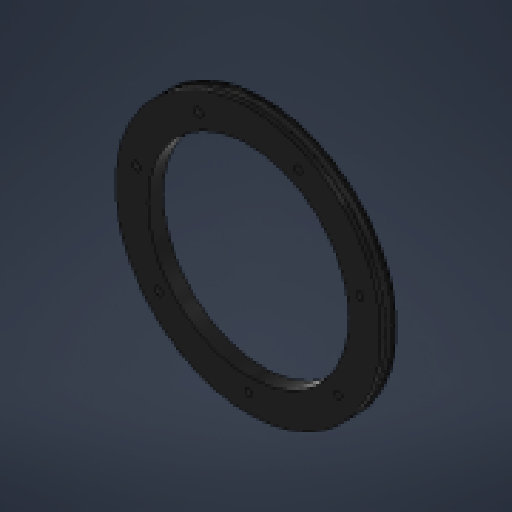
# Autodesk Inventor part: 3DPRINT,TURRET,BEARING,INNER
Saved by Autodesk Inventor 2026.1 (Build 301233020, 233B)
## iProperties
Created: 2026-02-09
Part Number: 3DPRINT,TURRET,BEARING,INNER
Material: Nylon 6/6
Document SubType Name: Modeling
Designer: littl
Density: 1.13 g/cm^3
Appearance: Smooth - Black
Mass: 187.156 g
Surface Area: 455.274 cm^2
Volume: 165.625 cm^3
Author: littl
Autodesk Inventor part; units mm, degrees
ref_plane "YZ Plane" through (0, 0, 0) normal (1, 0, 0) x (0, 1, 0)
ref_plane "XZ Plane" through (0, 0, 0) normal (0, 1, 0) x (-1, 0, 0)
ref_plane "XY Plane" through (0, 0, 0) normal (0, 0, 1) x (1, 0, 0)
sketch "Sketch1" plane through (0, 0, 0) normal (1, 0, 0) x (0, 1, 0)
  arc A0 (-107.5189, 2.6268) -> (-107.5189, -2.6268) centre (-105.3147, 0) ccw construction
  line L0 (-105.5687, 3.175) -> (-105.5687, -3.175) construction
  line L1 (-107.5189, 2.6268) -> (-107.5189, 4.635) construction
  line L2 (-106.3625, 5.1846) -> (-106.3625, 3.5971) construction
  line L3 (-107.5189, 2.6268) -> (-106.3625, 3.5971) construction
  line L4 (-107.5189, -2.6268) -> (-106.3625, -3.5971) construction
  line L5 (-131.7625, 5.1846) -> (-131.7625, -5.1846) construction
  line L6 (-131.7625, 5.1846) -> (-106.3625, 5.1846) construction
  line L7 (-131.7625, -5.1846) -> (-106.3625, -5.1846) construction
  line L8 (-106.3625, -5.1846) -> (-106.3625, -3.5971) construction
  circle A1 centre (-105.5687, 0) radius 3.175 construction
  line L9 (-35.1032, 0) -> (87.3968, 0) construction
  line L10 (-104.775, 5.1846) -> (-104.775, 3.5971)
  line L11 (-104.775, -5.1846) -> (-104.775, -3.5971)
  line L12 (-103.6186, 2.6268) -> (-104.775, 3.5971)
  line L13 (-103.6186, -2.6268) -> (-104.775, -3.5971)
  arc A2 (-103.6186, -2.6268) -> (-103.6186, 2.6268) centre (-105.8227, 0) ccw
  line L14 (-79.375, 5.1846) -> (-79.375, -5.1846)
  line L15 (0, -7.2584) -> (0, 7.2584) construction
  line L16 (-79.375, -5.1846) -> (-104.775, -5.1846)
  line L17 (-79.375, 5.1846) -> (-104.775, 5.1846) construction
  line L18 (-104.775, 5.1846) -> (-104.775, 8.5314)
  line L19 (-104.775, 8.5314) -> (-79.375, 8.5314)
  line L20 (-79.375, 8.5314) -> (-79.375, 5.1846)
  line L21 (-90.4875, 22.7342) -> (-90.4875, 8.5314) construction
  point P0 (0, 0)
  point P1 (0, 0)
  point P2 (-108.7437, 0)
  point P3 (-131.7625, 0)
  point P4 (-19.1031, 0)
  point P5 (0, 7.2584)
  point P6 (0, 0)
  point P7 (-143.7622, 15.4465)
  dimension "d0" = 6.35
  dimension "d1" = 3.429
  dimension "d2" = 50
  dimension "d3" = 1.5875
  dimension "d4" = 1.5875
  dimension "d5" = 158.75
  dimension "d7" = 25.4
  dimension "d8" = 25.4
  dimension "d9" = 180.975
  dimension "d23" = 13.716
  constraints: 42 end point, 8 point on circle, 8 symmetric about line, 5 perpendicular, 5 vertical, 4 point on line, 3 centre point, 3 midpoint, 2 collinear, 2 horizontal alignment, 2 parallel, 2 tangent, 2 vertical alignment, 1 coincident, 1 horizontal, 6 other
  measures "d0" diameter of A1
  measures "d1" radius of A0
  measures "d2" angle of L3 L1
  measures "d3" distance of L7.end L4.end
  measures "d4" distance between parallel lines of L10 L2
  measures "d7" distance of L18.end L19.end
  measures "d8" distance of L5.start L2.start
  measures "d23" distance between parallel lines of L16 L19
revolve "Revolution1" add sketch "Sketch1" angle 360 about axis through (0, 0, -7.2584) along (0, 0, 1)
sketch "Sketch2" plane through (0, 0, 8.5314) normal (0, 0, 1) x (1, 0, 0)
  point P0 (0, 0)
  point P1 (0, -90.4875)
  point P2 (70.746, -56.418)
  point P3 (88.2188, 20.1354)
  point P4 (39.2611, 81.5264)
  point P5 (-39.2611, 81.5264)
  point P6 (-88.2188, 20.1354)
  point P7 (-70.746, -56.418)
  dimension "d11" = 90.4875
  dimension "d14" = 360
  constraints: 1 vertical alignment, 8 other
  measures "d11" distance of point (0, 0) point (0, -90.487)
hole "Hole1" at (0, -90.4875, 8.5314) at (70.746, -56.418, 8.5314) at (88.2188, 20.1354, 8.5314) at (39.2611, 81.5264, 8.5314) at (-39.2611, 81.5264, 8.5314) at (-88.2188, 20.1354, 8.5314) at (-70.746, -56.418, 8.5314) direction (0, 0, -1) diameter 6.12 end through all
thicken "Thicken1" operation cut thickness 0.7937 both sides no extend neighbours no toward (0, 0, 1) faces at (-83.7461, 35.7818, -5.1846)
thicken "Thicken2" operation cut thickness 0.9656 both sides no extend neighbours no toward (0, 0, -1) faces at (-83.7461, 35.7818, 8.5314)
sketch "Sketch3" plane through (0, 0, -4.3908) normal (0, 0, -1) x (-1, 0, 0)
  line L0 (-102.1893, -8.577) -> (-91.0599, 34.4572)
  line L1 (-91.0599, 34.4572) -> (-78.7644, 31.2774)
  line L2 (-78.7644, 31.2774) -> (-89.8938, -11.7568)
  line L3 (-89.8938, -11.7568) -> (-102.1893, -8.577)
  line L4 (-102.1893, -8.577) -> (-78.7644, 31.2774) construction
  line L5 (-91.0599, 34.4572) -> (-89.8938, -11.7568) construction
  line L6 (72.9231, -53.8641) -> (84.0525, -10.83)
  line L7 (84.0525, -10.83) -> (96.3479, -14.0098)
  line L8 (96.3479, -14.0098) -> (85.2186, -57.0439)
  line L9 (85.2186, -57.0439) -> (72.9231, -53.8641)
  line L10 (72.9231, -53.8641) -> (96.3479, -14.0098) construction
  line L11 (84.0525, -10.83) -> (85.2186, -57.0439) construction
  line L12 (0, 0) -> (0, 27.097)
  point P0 (-90.4768, 11.3502)
  point P1 (84.6355, -33.9369)
  point P2 (-90.4768, 11.3502)
  point P3 (84.6355, -33.9369)
  point P4 (-90.4768, 11.3502)
  dimension "d28" = 44.45
  dimension "d29" = 12.7
  dimension "d30" = 14.5
  dimension "d31" = 91.186
  dimension "d32" = 91.186
  dimension "d33" = 11.3502
  constraints: 26 end point, 7 midpoint, 5 parallel, 2 equal length, 2 perpendicular, 1 collinear, 1 vertical
  measures "d28" distance of L1.end L2.end
  measures "d29" distance of L2.end L0.start
  measures "d30" angle of L2 L12
  measures "d31" distance of L12.start point (-90.477, 11.35)
  measures "d32" distance of point (84.636, -33.937) L12.start
  measures "d33" vertical distance of L12.start point (-90.477, 11.35)
extrude "Extrusion1" cut sketch "Sketch3" against normal blind 3.175
fillet "Fillet1" radius 6.35 8 edges at (78.7644, 31.2774, -2.8033) (91.0599, 34.4572, -2.8033) (102.1893, -8.577, -2.8033) (89.8938, -11.7568, -2.8033) (-84.0525, -10.83, -2.8033) (-72.9231, -53.8641, -2.8033) (-85.2186, -57.0439, -2.8033) (-96.3479, -14.0098, -2.8033)
equation "\"d8\" = d7"
equation "\"d32\" = d31"
body "Solid1"
